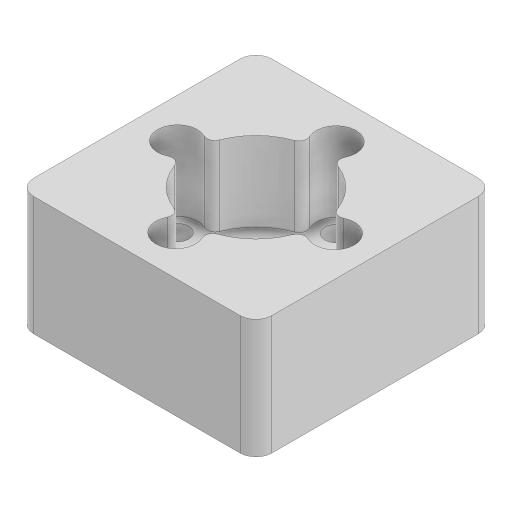
# Autodesk Inventor part: PDMS stretcher mould divided in parts
Saved by Autodesk Inventor 2023 (Build 270158000, 158)
## iProperties
Created: 2026-01-19
Part Number: PDMS stretcher mould divided in parts
Material: Generic
Document SubType Name: Modeling
Designer: ferrerx
Density: 1 g/cm^3
Appearance: Default
Author: ferrerx
Autodesk Inventor part; units mm, degrees
ref_plane "YZ Plane" through (0, 0, 0) normal (1, 0, 0) x (0, 1, 0)
ref_plane "XZ Plane" through (0, 0, 0) normal (0, 1, 0) x (-1, 0, 0)
ref_plane "XY Plane" through (0, 0, 0) normal (0, 0, 1) x (1, 0, 0)
sketch "Sketch1" plane through (0, 0, 0) normal (0, 1, 0) x (-1, 0, 0)
  line L0 (-15, 15) -> (15, 15)
  line L1 (15, 15) -> (15, -15)
  line L2 (15, -15) -> (-15, -15)
  line L3 (-15, -15) -> (-15, 15)
  line L4 (-15, 15) -> (15, -15) construction
  line L5 (15, 15) -> (-15, -15) construction
  point P0 (0, 0)
  dimension "d0" = 30
  dimension "d1" = 30
  constraints: 12 end point, 2 midpoint, 2 parallel, 1 horizontal, 1 perpendicular
  measures "d0" distance of L1.end L2.end
  measures "d1" distance of L0.end L1.end
extrude "Extrusion1" add sketch "Sketch1" along normal blind 5
sketch "Sketch2" plane through (0, 5, 0) normal (0, 1, 0) x (1, 0, 0)
  circle A0 centre (0, 0) radius 7
  dimension "d4" = 14
  constraints: 1 centre point, 1 coincident
  measures "d4" diameter of A0
extrude "Extrusion2" add sketch "Sketch2" along normal blind 10
sketch "Sketch3" plane through (0, 5, 0) normal (0, 1, 0) x (1, 0, 0)
  line L0 (-15, -15) -> (15, -15) projected
  line L1 (0, -15) -> (0, 15) construction
  line L2 (15, 15) -> (-15, 15) projected
  line L3 (0, 0.1067) -> (-10, 0.1067) construction
  circle A0 centre (-10, 0.1067) radius 1.425
  point P0 (0, 0)
  point P1 (0, 0)
  dimension "d7" = 2.85
  dimension "d8" = 10
  constraints: 4 end point, 3 midpoint, 1 centre point, 1 coincident, 1 horizontal, 1 point on line
  measures "d7" diameter of A0
  measures "d8" horizontal distance of point (0, 0) A0.centre
extrude "Extrusion3" add sketch "Sketch3" along normal blind 10
pattern_circular "Circular Pattern1" count 4 over 360 about axis through (0, 5, 0) along (0, 1, 0) of "Extrusion3"
sketch "Sketch4" plane through (0, 5, 0) normal (0, 1, 0) x (1, 0, 0)
  circle A0 centre (-10, 0.1067) radius 1.425 projected
  circle A1 centre (-10, 0.1067) radius 2.5
  circle A2 centre (0.1067, 10) radius 1.425 projected
  circle A3 centre (0.1067, 10) radius 2.5
  circle A4 centre (-0.1067, -10) radius 1.425 projected
  circle A5 centre (-0.1067, -10) radius 2.5
  circle A6 centre (10, -0.1067) radius 1.425 projected
  circle A7 centre (10, -0.1067) radius 2.5
  circle A8 centre (0, 0) radius 7 projected
  circle A9 centre (0, 0) radius 8
  line L0 (15, -15) -> (-15, -15)
  line L1 (-15, -15) -> (-15, 15)
  line L2 (-15, 15) -> (15, 15)
  line L3 (15, 15) -> (15, -15)
  line L4 (15, -15) -> (-15, 15) construction
  line L5 (-15, -15) -> (15, 15) construction
  point P0 (7.8729, -1.4203)
  point P1 (1.2519, -7.9014)
  point P2 (-1.4203, -7.8729)
  point P3 (-7.9014, -1.2519)
  point P4 (-7.8729, 1.4203)
  point P5 (-1.2519, 7.9014)
  point P6 (1.4203, 7.8729)
  point P7 (7.9014, 1.2519)
  dimension "d14" = 5
  dimension "d15" = 5
  dimension "d16" = 5
  dimension "d17" = 5
  dimension "d18" = 16
  constraints: 12 end point, 5 centre point, 5 coincident, 2 midpoint, 2 parallel, 1 horizontal, 1 perpendicular
  measures "d14" diameter of A1
  measures "d15" diameter of A5
  measures "d16" diameter of A3
  measures "d17" diameter of A7
  measures "d18" diameter of A9
extrude "Extrusion4" add sketch "Sketch4" along normal up to surface (10 mm away) contours L0 L1 L2 L3
fillet "Fillet1" radius 1 8 edges at (-1.2519, 10, -7.9014) (-7.8729, 10, -1.4203) (-7.9014, 10, 1.2519) (-1.4203, 10, 7.8729) (1.2519, 10, 7.9014) (7.8729, 10, 1.4203) (7.9014, 10, -1.2519) (1.4203, 10, -7.8729)
fillet "Fillet2" radius 2 4 edges at (15, 7.5, 15) (15, 7.5, -15) (-15, 7.5, 15) (-15, 7.5, -15)
sketch "Sketch5" plane through (-10, 15, -0.1067) normal (0, 1, 0) x (1, 0, 0)
  circle A0 centre (0, 0) radius 1.425
  circle A1 centre (0, 0) radius 1.425 projected
  point P0 (10, -0.1067)
  constraints: 2 concentric, 1 centre point
extrude "Extrusion5" cut sketch "Sketch5" against normal blind 20.5
pattern_circular "Circular Pattern2" count 4 over 360 about axis through (0, 5, 0) along (0, 1, 0) of "Extrusion5"
sketch "Sketch6" plane through (0, 15, 0) normal (0, 1, 0) x (1, 0, 0)
  circle A0 centre (0, 0) radius 7
  dimension "d28" = 14
  constraints: 1 centre point, 1 coincident
  measures "d28" diameter of A0
extrude "Extrusion6" cut sketch "Sketch6" against normal up to surface (10 mm away)
sketch "Sketch7" plane through (0, 5, 0) normal (0, 1, 0) x (1, 0, 0)
  circle A0 centre (0, 0) radius 1.45
  dimension "d31" = 2.9
  constraints: 1 centre point, 1 coincident
  measures "d31" diameter of A0
extrude "Extrusion7" cut sketch "Sketch7" against normal blind 10
equation "\"d1\" = d0"
equation "\"d15\" = d14"
equation "\"d16\" = d14"
equation "\"d17\" = d14"
body "Solid1"
